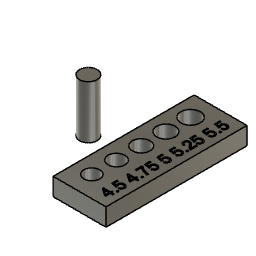
plate_holes (Autodesk Fusion 360 design; units mm, degrees)
Autodesk Fusion 360 part; units mm, degrees
sketch "Sketch1" plane through (0, 0, 0) normal (0, 0, 1) x (1, 0, 0)
  circle A0 centre (0, -7) radius 2.375
  circle A1 centre (0, 7) radius 2.625
  circle A2 centre (0, -14) radius 2.25
  circle A3 centre (0, 14) radius 2.75
  circle A4 centre (0, 0) radius 2.5
  line L0 (5, 20) -> (5, -20)
  line L1 (5, -20) -> (-5, -20)
  line L2 (-5, -20) -> (-5, 20)
  line L3 (-5, 20) -> (5, 20)
  dimension "d3" = 4.75
  dimension "d4" = 5.25
  dimension "d5" = 4.5
  dimension "d6" = 5.5
  dimension "d7" = 5
  constraint coincident A4.centre origin
  constraint vertical L0
  constraint perpendicular L0 L1
  constraint perpendicular L1 L2
  constraint perpendicular L0 L3
  measures "d3" diameter of A0
  measures "d4" diameter of A1
  measures "d5" diameter of A2
  measures "d6" diameter of A3
  measures "d7" diameter of A4
extrude "Extrude1" add sketch "Sketch1" along normal blind 5 makes body 1 in component "Component"
sketch "Sketch2" plane through (0, 0, 0) normal (0, 0, 1) x (1, 0, 0)
  circle A0 centre (-15, 0) radius 2.5
  dimension "d10" = 5
  measures "d10" diameter of A0
extrude "Extrude1'" add sketch "Sketch2" along normal blind 15 separate body makes body 2 in component "Component'"
extrude "Extrude2" add 1 faces at (5, 6.6667, 1.6667) along direction (1, 0, 0) blind 5 on bodies 1 bodies 1 in component "Component"
sketch "Sketch3" plane through (0, 0, 5) normal (0, 0, 1) x (-1, 0, 0)
  circle A0 centre (0, 14) radius 2.25
  circle A1 centre (0, 0) radius 2.5
  circle A2 centre (0, -7) radius 2.625
  circle A3 centre (0, 7) radius 2.375
  circle A4 centre (0, -14) radius 2.75
  line L0 (5, -20) -> (5, 20)
  line L1 (5, 20) -> (-10, 20)
  line L2 (-10, 20) -> (-10, -20)
  line L3 (-10, -20) -> (5, -20)
  line L4 (-8, 18) -> (-8, -18) construction
  line L5 (-8, -18) -> (-5, -18) construction
  line L6 (-5, -18) -> (-5, 18) construction
  line L7 (-5, 18) -> (-8, 18) construction
  dimension "d15" = 3
  text T0 "4.5 4.75 5 5.25 5.5" font "Arial" height 3 align centre middle in box 36 x 3 at (-8, 18) x (0, -1) y (1, 0) spacing 1
extrude "Extrude3" cut sketch "Sketch3" against normal blind 1 text T0 bodies 1 in component "Component"
component "Component" placed x (1, 0, 0) y (0, 1, 0) z (0, 0, 1) at (0, 0, 0)
component "Component'" placed x (1, 0, 0) y (0, 1, 0) z (0, 0, 1) at (0, 0, 0)
